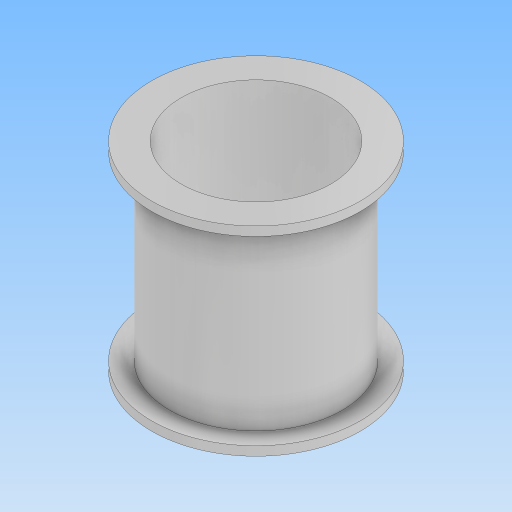
# Autodesk Inventor part: motor JS2622 jsumo
Saved by Autodesk Inventor 2023 (Build 270158000, 158)
## iProperties
Created: 2023-09-08
Part Number: motor JS2622 jsumo
Material: Generic
Document SubType Name: Modeling
Designer: MenMe
Density: 1 g/cm^3
Appearance: Default
Author: MenMe
Autodesk Inventor part; units mm, degrees
ref_plane "YZ Plane" through (0, 0, 0) normal (1, 0, 0) x (0, 1, 0)
ref_plane "XZ Plane" through (0, 0, 0) normal (0, 1, 0) x (-1, 0, 0)
ref_plane "XY Plane" through (0, 0, 0) normal (0, 0, 1) x (1, 0, 0)
sketch "Sketch1" plane through (0, 0, 0) normal (0, 0, 1) x (1, 0, 0)
  line L0 (0, 0) -> (0, 22)
  line L1 (0, 22) -> (11.5, 22)
  line L2 (11.5, 22) -> (11.5, 21)
  line L3 (11.5, 21) -> (9.5, 21)
  line L4 (9.5, 21) -> (9.5, 1)
  line L5 (9.5, 1) -> (11.5, 1)
  line L6 (11.5, 1) -> (11.5, 0)
  line L7 (11.5, 0) -> (0, 0)
  point P0 (5.75, 0)
  dimension "d0" = 22
  dimension "d1" = 20
  dimension "d2" = 1
  dimension "d3" = 23
  dimension "d4" = 19
  constraints: 16 end point, 6 perpendicular, 2 point on line, 1 midpoint, 1 vertical
  measures "d0" distance from line of point (5.75, 0) L1
  measures "d1" distance of L3.end L4.end
  measures "d2" distance of L5.end L6.end
  measures "d3" diameter of L1.end L0
  measures "d4" diameter of L4 L0
revolve "Revolution1" add sketch "Sketch1" angle 360 about axis through (0, 0, 0) along (0, 1, 0)
sketch "Sketch3" plane through (0, 22, 0) normal (0, 1, 0) x (1, 0, 0)
  circle A0 centre (0, 0) radius 8.25
  dimension "d6" = 16.5
  constraints: 1 centre point, 1 coincident
  measures "d6" diameter of A0
extrude "Extrusion1" cut sketch "Sketch3" against normal blind 16
sketch "Sketch4" plane through (0, 0, 0) normal (0, -1, 0) x (1, 0, 0)
  circle A0 centre (0, 0) radius 1.5
  dimension "d9" = 3
  constraints: 1 centre point, 1 coincident
  measures "d9" diameter of A0
extrude "Extrusion2" cut sketch "Sketch4" against normal through all
sketch "Sketch6" plane through (0, 0, 0) normal (1, 0, 0) x (0, 1, 0)
  circle A0 centre (3, 0) radius 1.5
  line L0 (0, -11.5) -> (0, 11.5) projected
  point P0 (0, 0)
  dimension "d13" = 3
  dimension "d14" = 3
  dimension "d15" = 3
  constraints: 1 centre point
  measures "d13" diameter of A0
  measures "d14" distance of point (0, 0) A0.centre
  measures "d15" distance from line of L0 A0.centre
extrude "Extrusion3" cut sketch "Sketch6" against normal blind 10
thread "Thread1" size "M3x0.5" class "6H" standard "ANSI Metric M Profile" full length
body "Solid1"
